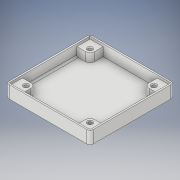
# Autodesk Inventor part: MD_kk_base_sa_1
Saved by Autodesk Inventor 2019 (Build 230136000, 136)
## iProperties
Created: 2019-02-28
Part Number: MD_kk_base_sa_1
Material: ABS プラスチック
Document SubType Name: Modeling
Designer: shun
Density: 1.06 g/cm^3
Appearance: 滑らか - 白
Author: shun
Autodesk Inventor part; units mm, degrees
ref_plane "YZ Plane" through (0, 0, 0) normal (1, 0, 0) x (0, 1, 0)
ref_plane "XZ Plane" through (0, 0, 0) normal (0, 1, 0) x (-1, 0, 0)
ref_plane "XY Plane" through (0, 0, 0) normal (0, 0, 1) x (1, 0, 0)
sketch "スケッチ1" plane through (0, 0, 0) normal (0, 1, 0) x (-1, 0, 0)
  line L0 (25, 25) -> (-25, 25) construction
  line L1 (-25, 25) -> (-25, -25) construction
  line L2 (-25, -25) -> (25, -25) construction
  line L3 (25, -25) -> (25, 25) construction
  line L4 (25, 25) -> (-25, -25) construction
  line L5 (-25, 25) -> (25, -25) construction
  line L6 (25.3, 25.3) -> (-25.3, 25.3)
  line L7 (-25.3, 25.3) -> (-25.3, -25.3)
  line L8 (-25.3, -25.3) -> (25.3, -25.3)
  line L9 (25.3, -25.3) -> (25.3, 25.3)
  line L10 (26.3, 26.3) -> (-26.3, 26.3)
  line L11 (-26.3, 26.3) -> (-26.3, -26.3)
  line L12 (-26.3, -26.3) -> (26.3, -26.3)
  line L13 (26.3, -26.3) -> (26.3, 26.3)
  line L14 (-20, 20) -> (20, 20) construction
  line L15 (20, 20) -> (20, -20) construction
  line L16 (20, -20) -> (-20, -20) construction
  line L17 (-20, -20) -> (-20, 20) construction
  line L18 (17, 25.3) -> (17, 20)
  arc A0 (17, 20) -> (20, 17) centre (20, 20) ccw
  line L19 (20, 17) -> (25.3, 17)
  line L20 (0, 0) -> (0, 25.3)
  line L21 (0, 25.3) -> (0, 26.3)
  line L22 (0, 0) -> (25.3, 0)
  line L23 (25.3, 0) -> (26.3, 0)
  dimension "d0" = 50
  dimension "d1" = 50
  dimension "d2" = 0.3
  dimension "d3" = 1
  dimension "d4" = 5
  dimension "d5" = 3
  constraints: 48 end point, 8 parallel, 6 midpoint, 6 perpendicular, 5 coincident, 4 point on line, 2 point on circle, 1 centre point, 1 horizontal, 9 other
  measures "d0" distance of L2.end L1.end
  measures "d1" distance of L1.end L0.end
  measures "d2" distance between parallel lines of L3 L9
  measures "d3" distance between parallel lines of L9 L13
  measures "d4" distance between parallel lines of L0 L14
  measures "d5" distance from line of L18 point (20, 20)
extrude "押し出し1" add sketch "スケッチ1" against normal blind 0.8 contours L9 L19 A0 L18 L6 | L6 L21 L10 L13 L23 L9 | L18 A0 L19 L9 L22 L20 L6
extrude "押し出し2" add sketch "スケッチ1" along normal blind 5.5 contours L9 L19 A0 L18 L6
extrude "押し出し3" add sketch "スケッチ1" along normal blind 1.5 and the other way blind 5.5 from surface at 5.5 contours L6 L21 L10 L13 L23 L9
hole "穴1" at (20, 0, 20) at (-20, 0, 20) at (-20, 0, -20) at (20, 0, -20) direction (0, -1, 0) diameter 2.5 end through all both
fillet "フィレット1" radius 0.5 1 edges at (-20, 5.5, 18.75)
mirror "ミラー1" about plane through (-26.3, 0, 0) normal (0, 0, -1) of "フィレット1", "穴1", "押し出し3", "押し出し2", "押し出し1"
mirror "ミラー2" about plane through (0, 0, 25.3) normal (1, 0, 0) of "フィレット1", "穴1", "押し出し3", "押し出し2", "押し出し1", "ミラー1"
fillet "フィレット2" radius 1 2 edges at (-25.3, 0, 0) (0, 0, 25.3)
fillet "フィレット3" radius 2 4 edges at (26.3, 3.1, 26.3) (-26.3, 3.1, 26.3) (-26.3, 3.1, -26.3) (26.3, 3.1, -26.3)
